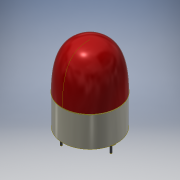
# Autodesk Inventor part: Circulina
Saved by Autodesk Inventor 2019 (Build 230136000, 136)
## iProperties
Created: 2019-06-20
Part Number: Circulina
Material: Steel, Mild, Welded
Document SubType Name: Modeling
Designer: hecto
Density: 7.85 g/cm^3
Appearance: Weld - Steel Mild
Author: hecto
Autodesk Inventor part; units mm, degrees
ref_plane "YZ Plane" through (0, 0, 0) normal (1, 0, 0) x (0, 1, 0)
ref_plane "XZ Plane" through (0, 0, 0) normal (0, 1, 0) x (-1, 0, 0)
ref_plane "XY Plane" through (0, 0, 0) normal (0, 0, 1) x (1, 0, 0)
sketch "Sketch1" plane through (0, 0, 0) normal (0, 1, 0) x (-1, 0, 0)
  circle A0 centre (0, 0) radius 45
  dimension "d0" = 90
  constraints: 1 centre point
  measures "d0" diameter of A0
extrude "Extrusion1" add sketch "Sketch1" along normal blind 50
sketch "Sketch2" plane through (0, 0, 0) normal (1, 0, 0) x (0, 1, 0)
  line L0 (50, -45) -> (50, 45) projected
  line L1 (50, 45) -> (50.7071, 45.7071)
  line L2 (50.7071, 45.7071) -> (90, 45) construction
  line L3 (90, 45) -> (126, 40) construction
  line L4 (126, 40) -> (125, 0) construction
  spline S0 degree 3 poles (50.7071, 45.7071) (90, 45) (126, 40) (125, 0) knots 1 1 1 1 2 2 2 2
  line L5 (125, 0) -> (50, 0)
  line L6 (50, 0) -> (50, 45)
  point P0 (0, 0)
  dimension "d3" = 1
  dimension "d4" = 135
  dimension "d5" = 40
  dimension "d6" = 76
  dimension "d7" = 75
  dimension "d8" = 40
  dimension "d9" = 45
  constraints: 6 end point, 1 collinear, 1 horizontal, 1 horizontal alignment, 1 midpoint, 3 other
  measures "d3" distance of L0.end L1.end
  measures "d4" angle of L0 L1
  measures "d5" distance from line of L0 L2.end
  measures "d6" distance from line of L0 L3.end
  measures "d7" distance from line of L0 L4.end
  measures "d8" vertical distance of L5.end L3.end
  measures "d9" vertical distance of L5.end L2.end
revolve "Revolution1" add sketch "Sketch2" angle 360 about axis through (0, 125, 0) along (0, -1, 0)
fillet "Fillet1" radius 2.3 2 edges at (31.8198, 50, -31.8198) (-31.8198, 50, 31.8198)
sketch "Sketch3" plane through (0, 0, 0) normal (0, -1, 0) x (1, 0, 0)
  line L0 (34.641, 0) -> (-17.3205, 30) construction
  line L1 (-17.3205, 30) -> (-17.3205, -30) construction
  line L2 (-17.3205, -30) -> (34.641, 0) construction
  circle A0 centre (0, 0) radius 34.641 construction
  circle A1 centre (-17.3205, 30) radius 6.25
  circle A2 centre (34.641, 0) radius 6.25
  circle A3 centre (-17.3205, -30) radius 6.25
  point P0 (-17.3205, 0)
  dimension "d12" = 60
  dimension "d13" = 12.5
  constraints: 6 end point, 5 coincident, 4 centre point, 2 equal length, 2 equal radius, 2 horizontal alignment, 2 point on circle, 1 midpoint
  measures "d12" distance of L1.end L0.start
  measures "d13" diameter of A1
extrude "Extrusion2" add sketch "Sketch3" along normal blind 5
sketch "Sketch4" plane through (-17.3205, -5, 30) normal (0, -1, 0) x (1, 0, 0)
  circle A0 centre (0, 0) radius 6.25 projected
  circle A1 centre (0, 0) radius 1.5
  point P0 (17.3205, -30)
  dimension "d16" = 3
  constraints: 1 centre point, 1 coincident
  measures "d16" diameter of A1
extrude "Extrusion3" add sketch "Sketch4" along normal blind 15 contours A1
chamfer "Chamfer1" distance 0.5 angle 45 1 edges at (-18.8205, -20, 30)
thread "Thread1" size "M3x0.5" class "6g" standard "ISO Metric profile" full length
pattern_circular "Circular Pattern1" count 3 over 360 about axis through (0, 0, 0) along (0, 1, 0) of "Extrusion3", "Chamfer1"
body "Solid1"
